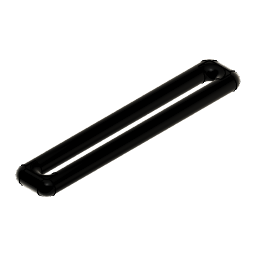
Rubber_22x4mm (Autodesk Fusion 360 design; units mm, degrees)
Autodesk Fusion 360 part; units mm, degrees
sketch "Sketch1" plane through (0, 0, 0) normal (0, 0, 1) x (1, 0, 0)
  line L0 (2, 11) -> (-2, 11)
  line L1 (-2, 11) -> (-2, -11)
  line L2 (-2, -11) -> (2, -11)
  line L3 (2, -11) -> (2, 11)
  line L4 (2, 11) -> (-2, -11) construction
  line L5 (-2, 11) -> (2, -11) construction
  line L6 (0.5, -9.5) -> (0.5, 9.5)
  line L7 (0.5, 9.5) -> (-0.5, 9.5)
  line L8 (-0.5, 9.5) -> (-0.5, -9.5)
  line L9 (-0.5, -9.5) -> (0.5, -9.5)
  dimension "d1" = 4
  dimension "d2" = 22
  dimension "d3" = -1.5
  constraint horizontal L0
  constraint perpendicular L0 L1
  constraint parallel L0 L2
  constraint parallel L1 L3
  constraint coincident L4 origin
  constraint coincident L5 origin
  measures "d1" distance of L1.end L2.end
  measures "d2" distance of L0.end L1.end
extrude "Extrude1" add sketch "Sketch1" along normal blind 1.5
fillet "Fillet1" radius 1 4 edges at (2, 11, 0.75) (-2, -11, 0.75) (2, -11, 0.75) (-2, 11, 0.75)
fillet "Fillet1" radius 0.5 4 edges at (-0.5, 9.5, 0.75) (0.5, 9.5, 0.75) (0.5, -9.5, 0.75) (-0.5, -9.5, 0.75)
fillet "Fillet2" radius 0.75 24 edges at (-1.7071, -10.7071, 1.5) (-2, 0, 1.5) (-1.7071, 10.7071, 1.5) (0, 11, 1.5) (1.7071, 10.7071, 1.5) (2, 0, 1.5) (1.7071, -10.7071, 1.5) (0, -11, 1.5) (0, 9.5, 1.5) (-0.5, 0, 1.5) (0, -9.5, 1.5) (0.5, 0, 1.5) (0, 11, 0) (-1.7071, 10.7071, 0) (-2, 0, 0) (-1.7071, -10.7071, 0) (0, -11, 0) (1.7071, -10.7071, 0) (2, 0, 0) (1.7071, 10.7071, 0) (0, 9.5, 0) (0.5, 0, 0) (0, -9.5, 0) (-0.5, 0, 0)
named bodies: "Rubber_22x4mm"
